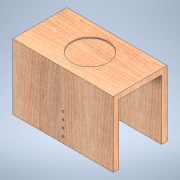
# Autodesk Inventor part: woodBracketForCamera
Saved by Autodesk Inventor 2022.2 (Build 262287000, 287)
## iProperties
Created: 2022-01-20
Part Number: woodBracketForCamera
Material: Wood (Birch)
Document SubType Name: Modeling
Designer: robst
Density: 0.55 g/cm^3
Appearance: Birch - Natural Polished
Author: robst
Autodesk Inventor part; units mm, degrees
ref_plane "YZ Plane" through (0, 0, 0) normal (1, 0, 0) x (0, 1, 0)
ref_plane "XZ Plane" through (0, 0, 0) normal (0, 1, 0) x (-1, 0, 0)
ref_plane "XY Plane" through (0, 0, 0) normal (0, 0, 1) x (1, 0, 0)
sketch "Sketch1" plane through (0, 0, 0) normal (0, 1, 0) x (-1, 0, 0)
  line L0 (174.625, 74.6125) -> (-174.625, 74.6125)
  line L1 (-174.625, 74.6125) -> (-174.625, -74.6125)
  line L2 (-174.625, -74.6125) -> (174.625, -74.6125)
  line L3 (174.625, -74.6125) -> (174.625, 74.6125)
  line L4 (174.625, 74.6125) -> (-174.625, -74.6125) construction
  line L5 (-174.625, 74.6125) -> (174.625, -74.6125) construction
  point P0 (0, 0)
  dimension "d0" = 149.225
  dimension "d4" = 349.25
  constraints: 12 end point, 2 midpoint, 2 parallel, 1 horizontal, 1 perpendicular
  measures "d0" distance of L1.end L0.end
  measures "d4" distance of L0.start L0.end
extrude "Extrusion1" add sketch "Sketch1" against normal blind 19.05
sketch "Sketch3" plane through (-174.625, 0, 74.6125) normal (0, 0, 1) x (1, 0, 0)
  line L0 (0, 0) -> (349.25, 0) projected
  line L1 (0, 0) -> (0, -19.05) projected
  line L2 (349.25, 0) -> (349.25, -19.05) projected
  line L3 (0, 0) -> (349.25, 0)
  line L4 (349.25, 0) -> (349.25, -228.6)
  line L5 (349.25, -228.6) -> (0, -228.6)
  line L6 (0, -228.6) -> (0, 0)
  point P0 (174.625, 0)
  dimension "d5" = 228.6
  constraints: 8 end point, 2 parallel, 1 horizontal, 1 perpendicular
  measures "d5" distance of L5.end L0.start
extrude "Extrusion2" add sketch "Sketch3" along normal blind 19.05
mirror "Mirror1" about plane through (0, 0, 0) normal (0, 0, 1) of "Extrusion2"
sketch "Sketch4" plane through (-174.625, 0, 93.6625) normal (0, 0, 1) x (1, 0, 0)
  line L0 (174.625, 0) -> (174.625, -228.6) construction
  line L1 (0, -228.6) -> (349.25, -228.6) construction
  point P0 (174.625, -207.6224)
  constraints: 2 end point, 1 midpoint, 1 point on line
hole "Hole1" at (0, -207.6224, 93.6625) direction (0, 0, -1) diameter 6.7564 end through all clearance for "Flat Head Machine Screw (82)" size "1/4" standard "Ansi Unified Screw Threads"
pattern_linear "Rectangular Pattern1" count 4 spacing 25.4 along (0, 1, 0) of "Hole1"
sketch "Sketch5" plane through (0, 0, 0) normal (0, 1, 0) x (1, 0, 0)
  circle A0 centre (0, 0) radius 63.5
  dimension "d18" = 127
  constraints: 1 centre point, 1 coincident
  measures "d18" diameter of A0
extrude "Extrusion3" cut sketch "Sketch5" against normal blind 2.54
equation "\"d0\" = widthTopBoard"
equation "\"d4\" = lengthTopBoard"
equation "\"d1\" = woodThickness"
equation "\"d6\" = woodThickness"
equation "\"widthTopBoard\" = 149.225"
equation "\"lengthTopBoard\" = 349.25"
equation "\"woodThickness\" = 19.05"
body "Solid1"
